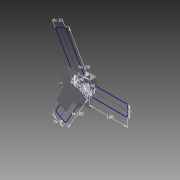
# Autodesk Inventor part: core
Saved by Autodesk Inventor 2015 (Build 190159000, 159)
## iProperties
Created: 2015-09-25
Part Number: core
Material: Generic
Document SubType Name: Modeling
Designer: Brian
Density: 1 g/cm^3
Appearance: Default
Author: Brian
Autodesk Inventor part; units mm, degrees
ref_plane "YZ Plane" through (0, 0, 0) normal (1, 0, 0) x (0, 1, 0)
ref_plane "XZ Plane" through (0, 0, 0) normal (0, 1, 0) x (-1, 0, 0)
ref_plane "XY Plane" through (0, 0, 0) normal (0, 0, 1) x (1, 0, 0)
sketch "Sketch1" plane through (0, 0, 0) normal (0, 1, 0) x (-1, 0, 0)
  line L0 (34.697, 0) -> (-17.3485, -30.0485)
  line L1 (-17.3485, -30.0485) -> (-17.3485, 30.0485)
  line L2 (-17.3485, 30.0485) -> (34.697, 0)
  line L3 (12.7, -12.7) -> (-12.7, -12.7) construction
  line L4 (-12.7, -12.7) -> (-12.7, 12.7) construction
  line L5 (-12.7, 12.7) -> (12.7, 12.7) construction
  line L6 (12.7, 12.7) -> (12.7, -12.7) construction
  line L7 (-17.3485, 15) -> (-117.3485, 15)
  line L8 (-117.3485, 15) -> (-117.3485, -15)
  line L9 (-117.3485, -15) -> (-17.3485, -15)
  line L10 (-4.3161, -22.5243) -> (45.6839, -109.1268)
  line L11 (45.6839, -109.1268) -> (71.6646, -94.1268)
  line L12 (71.6646, -94.1268) -> (21.6646, -7.5243)
  line L13 (0, 0) -> (58.6743, -101.6268) construction
  line L14 (0, 0) -> (-117.3485, 0) construction
  line L15 (-4.3161, 22.5243) -> (45.6839, 109.1268)
  line L16 (45.6839, 109.1268) -> (71.6646, 94.1268)
  line L17 (71.6646, 94.1268) -> (21.6646, 7.5243)
  line L18 (58.6743, 101.6268) -> (0, 0) construction
  line L19 (11.5, -11.5) -> (-11.5, -11.5)
  line L20 (-11.5, -11.5) -> (-11.5, 11.5)
  line L21 (-11.5, 11.5) -> (11.5, 11.5)
  line L22 (11.5, 11.5) -> (11.5, -11.5)
  circle A0 centre (-12, 20.7846) radius 2.5
  line L23 (0, 0) -> (-17.3485, 30.0485) construction
  line L24 (0, 0) -> (-17.3485, -30.0485) construction
  line L25 (0, 0) -> (34.697, 0) construction
  circle A1 centre (-12, -20.7846) radius 2.5
  circle A2 centre (24, 0) radius 2.5
  dimension "d1" = 25.4
  dimension "d2" = 30
  dimension "d3" = 100
  dimension "d4" = 30
  dimension "d5" = 100
  dimension "d6" = 120
  dimension "d7" = 30
  dimension "d8" = 100
  dimension "d9" = 120
  dimension "d10" = 23
  dimension "d21" = 5
  dimension "d22" = 24
  dimension "d23" = 5
  dimension "d24" = 5
  dimension "d25" = 24
  dimension "d26" = 24
  constraints: 52 end point, 11 point on line, 5 perpendicular, 4 coincident, 4 parallel, 3 centre point, 3 midpoint, 2 horizontal, 2 horizontal alignment, 1 vertical, 25 other
  measures "d1" distance of L5.end L3.start
  measures "d2" distance of L7.end L8.end
  measures "d3" distance of L8.end L9.end
  measures "d4" distance of L10.end L11.end
  measures "d5" distance of L10.start L10.end
  measures "d6" angle of L14 L13
  measures "d7" distance of L15.end L16.end
  measures "d8" distance of L15.start L15.end
  measures "d9" angle of L14 L18
  measures "d10" distance of L21.end L19.start
  measures "d21" diameter of A0
  measures "d22" distance of point (0, 0) A0.centre
  measures "d23" diameter of A1
  measures "d24" diameter of A2
  measures "d25" distance of A1.centre point (0, 0)
  measures "d26" distance of point (0, 0) A2.centre
extrude "Extrusion1" add sketch "Sketch1" against normal blind 30 contours L0 L1 L2 | L12 L11 L10 L0 | L2 L15 L16 L17 | L9 L8 L7 L1 | L19 L20 L21 L22 | A0 | A1 | A2
sketch "Sketch2" plane through (17.3485, 0, 15) normal (0, 0, 1) x (1, 0, 0)
  line L0 (0, 0) -> (100, 0) construction
  line L1 (0, -30) -> (0, 0) construction
  line L2 (100, -30) -> (0, -30) construction
  line L3 (100, 0) -> (100, -30) projected
  line L4 (0, 0) -> (100, -83.91)
  line L5 (100, 0) -> (100, -30) projected
  line L6 (100, -83.91) -> (100, 0)
  line L7 (0, 0) -> (100, 0)
  point P0 (-17.3485, 0)
  dimension "d13" = 40
  constraints: 6 end point, 1 collinear, 1 perpendicular, 1 point on line
  measures "d13" angle of L4 L0
extrude "Extrusion2" cut sketch "Sketch2" against normal up to next
pattern_circular "Circular Pattern1" count 3 over 360 about axis through (0, -10, 0) along (0, 1, 0) of "Extrusion2"
extrude "Extrusion3" add sketch "Sketch1" along normal blind 25.4 contours L19 L20 L21 L22
extrude "Extrusion4" cut sketch "Sketch1" against normal up to next contours A0 | A1 | A2
equation "\"d4\" = d2"
equation "\"d5\" = d3"
equation "\"d7\" = d2"
equation "\"d8\" = d3"
equation "\"d9\" = d6"
equation "\"d23\" = d21"
equation "\"d24\" = d21"
equation "\"d25\" = d22"
equation "\"d26\" = d22"
body "Solid1"
